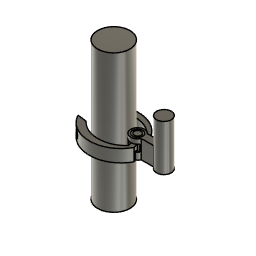
30mm pole to 16mm pole ziptie fastaner (Autodesk Fusion 360 design; units mm, degrees)
Autodesk Fusion 360 part; units mm, degrees
sketch "Sketch1" plane through (0, 0, 0) normal (0, 0, 1) x (1, 0, 0) in component "pole"
  circle A0 centre (0, 0) radius 17.5
  dimension "d1" = 35
  constraint coincident A0.centre origin
  measures "d1" diameter of A0
extrude "Extrude1" add sketch "Sketch1" along normal blind 150 makes body 1 in component "pole"
move_body "Move1" bodies 1 to x (1, 0, 0) y (0, 1, 0) z (0, 0, 1) at (0, 0, -55) in component "pole"
sketch "Sketch1 (2)" plane through (0, 0, 0) normal (0, 0, 1) x (1, 0, 0) in component "the thing"
  line L0 (18, 0) -> (26, 0) construction
  circle A0 centre (26, 0) radius 7.5
  circle A1 centre (26, 0) radius 3.75
  circle A2 centre (26, 0) radius 5.5
  dimension "d5" = 8
  constraint horizontal L0
  constraint coincident L0.end A0.centre
  constraint concentric A0 A1
  constraint concentric A1 A2
  measures "d5" distance of L0.start L0.end
extrude "Extrude1'" add sketch "Sketch1 (2)" along normal blind 20 separate body makes body 2 at (29.7453, -0.1869, 13.3333) makes body 3 at (33.4907, -0.3738, 13.3333) in component "the thing"
ref_plane "WorkPlane1" through (26, -7.5, 13.3774) normal (0, -1, 0) x (-1, 0, 0) in component "the thing"
sketch "Sketch4" plane through (0, -7.5, 0) normal (0, -1, 0) x (-1, 0, 0) in component "the thing"
  line L0 (-18.5, -15) -> (-33.5, -15)
  line L1 (-33.5, -15) -> (-33.5, -7.5)
  line L2 (-33.5, -7.5) -> (-18.5, -7.5)
  line L3 (-18.5, -7.5) -> (-18.5, -15)
  constraint horizontal L0
  constraint vertical L1
  constraint horizontal L2
  constraint vertical L3
extrude "Extrude6" cut sketch "Sketch4" against normal blind 3.5 bodies 3 in component "the thing"
ref_plane "WorkPlane2" through (26.9706, -3.6222, 8.9468) normal (0.258819, -0.965926, 0) x (-0.965926, -0.258819, 0) in component "the thing"
sketch "Sketch5" plane through (2.7122, -10.1222, 0) normal (0.258819, -0.965926, 0) x (-0.965926, -0.258819, 0) in component "the thing"
  line L0 (-22.5, -13.5) -> (-27.5, -13.5)
  line L1 (-27.5, -13.5) -> (-27.5, -8.5)
  line L2 (-27.5, -8.5) -> (-22.5, -8.5)
  line L3 (-22.5, -8.5) -> (-22.5, -13.5)
  dimension "d23" = 5
  dimension "d24" = 5
  constraint horizontal L0
  constraint vertical L1
  constraint horizontal L2
  constraint vertical L3
  measures "d23" distance of L0.start L0.end
  measures "d24" distance of L0.start L2.end
extrude "Extrude7" add sketch "Sketch5" against normal blind 2.5 bodies 2 in component "the thing"
move_face "OffsetFaces1" offset 6 1 faces at (25.2872, -4.0733, 11.8333) on bodies 2 in component "the thing"
fillet "Fillet2" radius 4 1 edges at (26.8218, -3.6588, 8.5) on bodies 2 in component "the thing"
sketch "Sketch6" plane through (0, 0, 8.5) normal (0, 0, -1) x (1, 0, 0) in component "the thing"
  arc A0 (30.2131, 6.5048) -> (25.3633, 7.7238) centre (26, 0) ccw
  line L0 (30.2131, 6.5048) -> (30.8281, 8.8003)
  line L1 (30.8281, 8.8003) -> (25.9985, 10.0943)
  line L2 (25.9985, 10.0943) -> (25.3633, 7.7238)
  line L3 (25.9985, 10.0943) -> (30.8281, 8.8003)
  line L4 (30.8281, 8.8003) -> (30.3622, 7.0616)
  line L5 (25.9985, 10.0943) -> (25.5326, 8.3557)
  line L6 (25.5326, 8.3557) -> (30.3622, 7.0616)
  line L7 (30.8281, 8.8003) -> (30.3622, 7.0616)
  line L8 (25.9985, 10.0943) -> (25.5326, 8.3557)
  line L9 (25.5326, 8.3557) -> (30.3622, 7.0616)
  line L10 (30.8281, 8.8003) -> (25.9985, 10.0943)
  dimension "d32" = 1.8
  dimension "d33" = 1.8
  constraint coincident L1.end L2.start
  constraint coincident L0.end L1.start
  constraint perpendicular L3 L4
  constraint coincident L2 L5.end
  measures "d32" distance of L0.end L4.end
  measures "d33" distance of L1.end L5.end
extrude "Extrude8" add sketch "Sketch6" along normal up to surface (8.5 mm away) contours L0 L1 L2 L3 L4 L5 L6 L7 L8 L9 L10 bodies 2 in component "the thing"
sketch "Sketch7" plane through (0, 0, 0) normal (0, 0, 1) x (1, 0, 0) in component "the thing"
  circle A0 centre (26, 0) radius 7.5 construction
  line L0 (30.8281, -8.8003) -> (30.8281, -5.7393) construction
  line L1 (30.8281, -5.7393) -> (30.8281, 5.7393) construction
  line L2 (30.8281, 5.7393) -> (30.8281, 8.8003) construction
  line L3 (25.9985, -10.0943) -> (25.9985, -7.5) construction
  line L4 (25.9985, -7.5) -> (25.9985, 7.5) construction
  line L5 (25.9985, 7.5) -> (25.9985, 10.094) construction
  point P0 (30.3622, -7.0616)
  point P1 (30.8281, -8.8003)
  point P2 (25.9985, -10.0943)
  dimension "d38" = 3.061
  dimension "d39" = 3.061
  dimension "d40" = 2.5943
  dimension "d41" = 2.594
  constraint vertical L0
  constraint coincident P1 L0.start
  constraint vertical L1
  constraint coincident A0 L1.end
  constraint vertical L2
  constraint vertical L3
  constraint coincident P2 L3.start
  constraint coincident A0 L4.end
  constraint parallel L3 L4
  constraint parallel L4 L5
  measures "d38" distance of P1 L0.end
  measures "d39" distance of L1.end L2.end
  measures "d40" distance of P2 L3.end
  measures "d41" distance of L4.end L5.end
sketch "Sketch8" plane through (0, 0, 0) normal (0, 0, 1) x (1, 0, 0) in component "the thing"
  arc A0 (-30, -8.8003) -> (30.8281, -8.8003) centre (0.4141, 7.508) ccw
  arc A1 (-20, -10.0943) -> (25.9985, -10.0943) centre (2.9992, 11.1989) ccw
  arc A2 (25.9985, 10.094) -> (-20, 10.094) centre (2.9992, -11.1982) ccw
  arc A3 (30.8281, 8.8003) -> (-30, 8.8003) centre (0.4141, -8.5731) ccw
  line L0 (-30, -8.8003) -> (-20, -10.0943)
  line L1 (-30, 8.8003) -> (-20, 10.094)
  line L2 (25.9985, -10.0943) -> (30.8281, -8.8003)
  line L3 (25.9985, 10.094) -> (30.8281, 8.8003)
  point P0 (30.8281, -8.8003)
  point P1 (25.9985, -10.0943)
  point P2 (25.9985, 10.094)
  point P3 (30.8281, 8.8003)
  constraint coincident P0 A0.end
  constraint coincident P1 A1.end
  constraint coincident P2 A2.start
  constraint tangent A2 A3
  constraint coincident P3 A3.start
sketch "Sketch9" plane through (0, 0, 0) normal (0, 0, 1) x (1, 0, 0) in component "the thing"
  line L0 (30.8281, 8.8003) -> (25.9985, 10.094)
  line L1 (30.8281, 5.7393) -> (25.9985, 7.5)
  line L2 (25.9985, 7.5) -> (25.9985, 10.094)
  line L3 (30.8281, 5.7393) -> (30.8281, 8.8003)
  point P0 (30.8281, 8.8003)
  point P1 (25.9985, 10.094)
  point P2 (30.8281, 5.7393)
  point P3 (25.9985, 7.5)
  constraint coincident P0 L0.start
  constraint coincident P1 L0.end
  constraint coincident P2 L1.start
  constraint coincident P3 L1.end
extrude "Extrude9" add sketch "Sketch9" along normal blind 13.5 bodies 3 in component "the thing"
extrude "Extrude10" add sketch "Sketch8" along normal blind 13.5 bodies 2 3 in component "the thing"
ref_plane "WorkPlane3" through (33.5, 0, 10.1602) normal (1, 0, 0) x (0, -1, 0) in component "the thing"
sketch "Sketch10" plane through (33.5, 0, 0) normal (1, 0, 0) x (0, 1, 0) in component "the thing"
  line L0 (-3, 20) -> (5, 20)
  line L1 (5, 20) -> (5, 0)
  line L2 (5, 0) -> (-3, 0)
  line L3 (-3, 0) -> (-3, 20)
  constraint horizontal L0
  constraint vertical L1
  constraint horizontal L2
  constraint vertical L3
extrude "Extrude11" add sketch "Sketch10" against normal blind 2 bodies 3 in component "the thing"
move_face "OffsetFaces2" offset 13 1 faces at (33.5, 0.6667, 6.6667) on bodies 3 in component "the thing"
sketch "Sketch11" plane through (0, 0, 0) normal (0, 0, 1) x (1, 0, 0) in component "the thing"
  line L0 (46.5, 5) -> (46.5, -3) construction
  line L1 (46.5, 1) -> (53.5, 1) construction
  circle A0 centre (53.5, 1) radius 8
  dimension "d54" = 7
  dimension "d55" = 16
  constraint midpoint L0 L1.start
  constraint perpendicular L0 L1
  constraint coincident L1.end A0.centre
  measures "d54" distance of L1.start L1.end
  measures "d55" diameter of A0
extrude "Extrude13" add sketch "Sketch11" along normal blind 50 bodies 3 in component "the thing"
sketch "Sketch1 (3)" plane through (0, 0, 0) normal (0, 1, 0) x (1, 0, 0)
  circle A0 centre (-22, -6.5) radius 5
  dimension "d59" = 10
  measures "d59" diameter of A0
extrude "Extrude14" cut sketch "Sketch1 (3)" along normal blind 54 from surface at -27 bodies 2 3 in component "the thing"
component "pole" placed x (1, 0, 0) y (0, 1, 0) z (0, 0, 1) at (0, 0, 0)
component "the thing" placed x (1, 0, 0) y (0, 1, 0) z (0, 0, 1) at (0, 0, 0)
